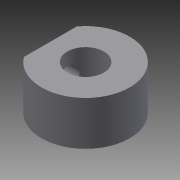
# Autodesk Inventor part: collar
Saved by Autodesk Inventor 2013 SP2 (Build 170200200, 200)
## iProperties
Created: 2016-03-08
Part Number: collar
Material: Generic
Document SubType Name: Modeling
Designer: 2016nriopell
Density: 1 g/cm^3
Author: 2016nriopell
Autodesk Inventor part; units mm, degrees
ref_plane "YZ Plane" through (0, 0, 0) normal (1, 0, 0) x (0, 1, 0)
ref_plane "XZ Plane" through (0, 0, 0) normal (0, 1, 0) x (-1, 0, 0)
ref_plane "XY Plane" through (0, 0, 0) normal (0, 0, 1) x (1, 0, 0)
sketch "Sketch1" plane through (0, 0, 0) normal (0, 1, 0) x (-1, 0, 0)
  circle A0 centre (0, 0) radius 12.7
  circle A1 centre (0, 0) radius 5.2705
  line L0 (12.7, 0) -> (10.16, 0)
  line L1 (10.16, 0) -> (10.16, 7.62)
  line L2 (10.16, 0) -> (10.16, -7.62)
  dimension "d0" = 25.4
  dimension "d1" = 10.541
  dimension "d4" = 2.54
  constraints: 6 end point, 3 point on circle, 2 centre point, 2 coincident, 1 collinear, 1 horizontal, 1 perpendicular
  measures "d0" diameter of A0
  measures "d1" diameter of A1
  measures "d4" distance of L0.start L0.end
extrude "Extrusion1" add sketch "Sketch1" against normal blind 12.7 contours L1 L2 A0
sketch "Sketch2" plane through (-10.16, 0, -7.62) normal (-1, 0, 0) x (0, 0, 1)
  circle A0 centre (7.62, -6.35) radius 2.7781
  point P0 (7.62, 0)
  dimension "d5" = 5.5563
  constraints: 1 centre point
  measures "d5" diameter of A0
extrude "Extrusion2" cut sketch "Sketch2" against normal blind 12.7
body "Solid1"
